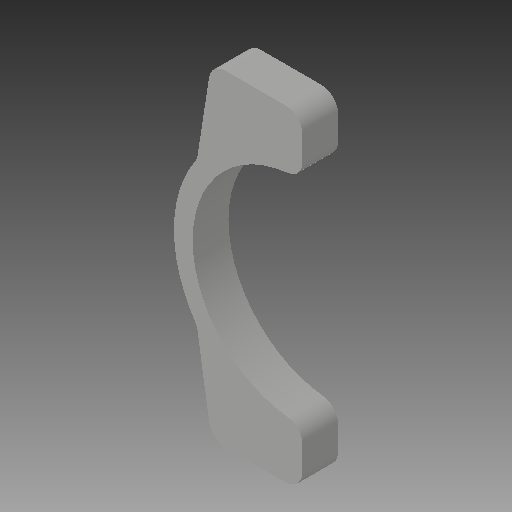
# Autodesk Inventor part: syringe_stopper
Saved by Autodesk Inventor 2019 (Build 230136000, 136)
## iProperties
Created: 2017-11-04
Part Number: syringe_stopper
Material: Generic
Document SubType Name: Modeling
Designer: MISAKA
Density: 1 g/cm^3
Appearance: Default
Author: MISAKA
Autodesk Inventor part; units mm, degrees
ref_plane "YZ Plane" through (0, 0, 0) normal (1, 0, 0) x (0, 1, 0)
ref_plane "XZ Plane" through (0, 0, 0) normal (0, 1, 0) x (-1, 0, 0)
ref_plane "XY Plane" through (0, 0, 0) normal (0, 0, 1) x (1, 0, 0)
sketch "Sketch1" plane through (0, 0, 0) normal (0, 0, 1) x (1, 0, 0)
  line L0 (-7.7822, 21) -> (3.6178, 21) projected
  line L1 (3.6178, 21) -> (20.2178, 21) projected
  line L2 (-7.7822, -21) -> (-7.7822, 21) projected
  line L3 (3.6178, -21) -> (-7.7822, -21) projected
  line L4 (3.6178, -21) -> (10.2178, -21) projected
  line L5 (10.2178, -21) -> (10.2178, -12.4061) projected
  arc A0 (17.6857, 12.5652) -> (17.6857, -12.5652) centre (14.2178, 0) ccw projected
  line L6 (10.2178, 21) -> (10.2178, 12.4061) projected
  line L7 (1.7178, 8.8712) -> (3.6178, 21) projected
  arc A1 (1.7178, 8.8712) -> (1.7178, -8.8712) centre (14.2178, 0) ccw projected
  line L8 (1.7178, -8.8712) -> (3.6178, -21) projected
  line L9 (10.2178, -21) -> (14.6178, -21)
  line L10 (14.6178, -21) -> (14.6178, -13.0289)
  line L11 (3.6178, 21) -> (14.6178, 21)
  line L12 (14.6178, 13.0289) -> (14.6178, 21)
  arc A2 (14.6178, 13.0289) -> (14.6178, -13.0289) centre (14.2178, 0) ccw
  point P0 (0, 0)
  dimension "d0" = 11
  constraints: 8 end point, 4 point on circle, 2 perpendicular, 1 centre point, 1 coincident, 1 collinear, 1 horizontal, 1 point on line
  measures "d0" distance from line of L10 L3.start
extrude "Extrusion1" add sketch "Sketch1" along normal blind 4.393 contours L1 L6 A0 L5 L4 L8 A1 L7 | L1 L12 A0 L6 | L5 A0 L10 L9
thicken "Thicken1" operation add thickness 1 both sides no extend neighbours yes toward (0, -1, 0) faces at (10.9511, 21, 1.4643)
thicken "Thicken2" operation add thickness 1 both sides no extend neighbours yes toward (0, 1, 0) faces at (7.2844, -21, 1.4643)
fillet "Fillet1" radius 2 8 edges at (14.6178, 13.0289, 2.1965) (14.6178, -20, 2.1965) (14.6178, 20, 2.1965) (3.4611, 20, 2.1965) (3.4611, -20, 2.1965) (1.7178, -8.8712, 2.1965) (1.7178, 8.8712, 2.1965) (14.6178, -13.0289, 2.1965)
body "Solid1"
